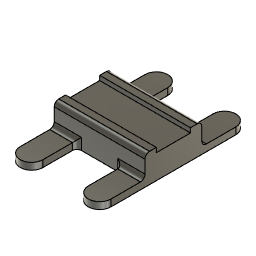
standoff for lid v3 (Autodesk Fusion 360 design; units mm, degrees)
Autodesk Fusion 360 part; units mm, degrees
sketch "Sketch1" plane through (0, 0, 0) normal (0, 0, 1) x (1, 0, 0)
  line L0 (20, -12.5) -> (-20, -12.5)
  line L1 (-20, -12.5) -> (-20, 12.5)
  line L2 (-20, 12.5) -> (20, 12.5)
  line L3 (20, 12.5) -> (20, -12.5)
  line L4 (20, -12.5) -> (-20, 12.5) construction
  line L5 (-20, -12.5) -> (20, 12.5) construction
  dimension "d1" = 40
  dimension "d2" = 25
  constraint horizontal L0
  constraint perpendicular L0 L1
  constraint parallel L0 L2
  constraint parallel L1 L3
  constraint coincident L4 origin
  constraint coincident L5 origin
  measures "d1" distance of L1.end L2.end
  measures "d2" distance of L0.end L1.end
extrude "Extrude1" add sketch "Sketch1" along normal blind 12.7
sketch "Sketch2" plane through (0, 0, 12.7) normal (0, 0, 1) x (-1, 0, 0)
  line L0 (-20, -12.5) -> (20, -12.5)
  line L1 (20, -12.5) -> (20, 12.5)
  line L2 (20, 12.5) -> (-20, 12.5)
  line L3 (-20, 12.5) -> (-20, -12.5)
  line L4 (-20, 7.5) -> (20, 7.5)
  line L5 (20, 7.5) -> (20, -7.5)
  line L6 (20, -7.5) -> (-20, -7.5)
  line L7 (-20, -7.5) -> (-20, 7.5)
  line L8 (-20, 7.5) -> (20, -7.5) construction
  line L9 (20, 7.5) -> (-20, -7.5) construction
  dimension "d5" = 40
  dimension "d6" = 15
  constraint horizontal L4
  constraint perpendicular L4 L5
  constraint parallel L4 L6
  constraint parallel L5 L7
  constraint coincident L8 origin
  constraint coincident L9 origin
  measures "d5" distance of L5.end L6.end
  measures "d6" distance of L4.end L5.end
extrude "Extrude2" cut sketch "Sketch2" against normal blind 2 contours L1 L3 L4 L5 L6 L7
sketch "Sketch3" plane through (0, -12.5, 0) normal (0, -1, 0) x (1, 0, 0)
  line L0 (-20, 0) -> (20, 0)
  line L1 (20, 0) -> (20, 12.7)
  line L2 (20, 12.7) -> (-20, 12.7)
  line L3 (-20, 12.7) -> (-20, 0)
  line L4 (0, 12.7) -> (0, 0) construction
  line L5 (20, 0) -> (10, 0)
  line L6 (10, 0) -> (10, 3)
  line L7 (10, 3) -> (20, 3)
  line L8 (20, 3) -> (20, 0)
  line L9 (-20, 0) -> (-10, 0)
  line L10 (-10, 0) -> (-10, 3)
  line L11 (-10, 3) -> (-20, 3)
  line L12 (-20, 3) -> (-20, 0)
  point P0 (0, 12.7)
  dimension "d23" = 10
  dimension "d24" = 3
  dimension "d25" = 10
  dimension "d26" = 3
  constraint midpoint L2 P0
  constraint coincident P0 L4.start
  constraint coincident L4.end origin
  constraint horizontal L5
  constraint vertical L6
  constraint horizontal L7
  constraint vertical L8
  constraint coincident L0.end L1.start
  constraint horizontal L9
  constraint vertical L10
  constraint horizontal L11
  constraint vertical L12
  constraint coincident L0.start L3.end
  measures "d23" distance of L0.end L5.end
  measures "d24" distance of L0.end L7.end
  measures "d25" distance of L0.start L9.end
  measures "d26" distance of L0.start L11.end
extrude "Extrude5" add sketch "Sketch3" along normal blind 20 contours L0 L3 L9 L10 L11 L12 | L0 L1 L5 L6 L7 L8
sketch "Sketch6" plane through (0, 12.5, 0) normal (0, 1, 0) x (-1, 0, 0)
  line L0 (-20, 0) -> (20, 0)
  line L1 (20, 0) -> (20, 12.7)
  line L2 (20, 12.7) -> (-20, 12.7)
  line L3 (-20, 12.7) -> (-20, 0)
  line L4 (-10, 3) -> (-20, 3)
  line L5 (-10, 0) -> (-10, 3)
  line L6 (-20, 0) -> (-10, 0)
  line L7 (-20, 3) -> (-20, 0)
  line L8 (10, 0) -> (10, 3)
  line L9 (10, 3) -> (20, 3)
  line L10 (20, 0) -> (10, 0)
  line L11 (20, 3) -> (20, 0)
  line L12 (-20, 0) -> (-10, 0)
  line L13 (-10, 0) -> (-10, 3)
  line L14 (-10, 3) -> (-20, 3)
  line L15 (-20, 3) -> (-20, 0)
  line L16 (20, 0) -> (10, 0)
  line L17 (10, 0) -> (10, 3)
  line L18 (10, 3) -> (20, 3)
  line L19 (20, 3) -> (20, 0)
  constraint horizontal L12
  constraint vertical L13
  constraint horizontal L14
  constraint vertical L15
  constraint coincident L4.start L5.end
  constraint coincident L0.start L3.end
  constraint horizontal L16
  constraint vertical L17
  constraint horizontal L18
  constraint vertical L19
  constraint coincident L8.end L9.start
  constraint coincident L0.end L1.start
extrude "Extrude6" add sketch "Sketch6" along normal blind 20 contours L0 L3 L4 L5 L6 L7 L12 L13 L14 L15 | L0 L1 L8 L9 L10 L11 L16 L17 L18 L19
fillet "Fillet5" radius 2 10 edges at (-10, 12.5, 1.5) (-15, 12.5, 3) (15, 12.5, 3) (0, 12.5, 12.7) (0, -12.5, 12.7) (10, 12.5, 1.5) (-15, -12.5, 3) (10, -12.5, 1.5) (15, -12.5, 3) (-10, -12.5, 1.5)
fillet "Fillet6" radius 5 8 edges at (-20, -32.5, 1.5) (-10, -32.5, 1.5) (10, -32.5, 1.5) (20, -32.5, 1.5) (-10, 32.5, 1.5) (20, 32.5, 1.5) (-20, 32.5, 1.5) (10, 32.5, 1.5)
equation "d3 = 25.4 mm / 2"
equation "d25 = d23"
equation "d26 = d24"
